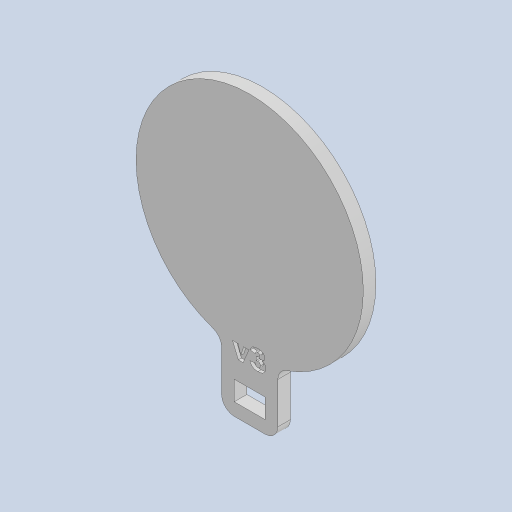
# Autodesk Inventor part: door_03
Saved by Autodesk Inventor 2024.4 (Build 284460030, 460C)
## iProperties
Created: 2026-07-13
Part Number: door_03
Material: Generic
Document SubType Name: Modeling
Designer: tooles01
Density: 1 g/cm^3
Appearance: Default
d0: 36.000 mm
d3: 4.900 mm
d4: 3.200 mm
d5: 10.000 mm
d6: 2.000 mm
d7: 2.000 mm
door_diameter: 36.000 mm
handle_height: 10.000 mm
spacing_height: 2.000 mm
spacing_width: 2.000 mm
axle_height: 3.100 mm
axle_width: 4.900 mm
x_e1: 0.00 deg
door_thickness: 2.000 mm
Author: tooles01
Autodesk Inventor part; units mm, degrees
ref_plane "YZ Plane" through (0, 0, 0) normal (1, 0, 0) x (0, 1, 0)
ref_plane "XZ Plane" through (0, 0, 0) normal (0, 1, 0) x (-1, 0, 0)
ref_plane "XY Plane" through (0, 0, 0) normal (0, 0, 1) x (1, 0, 0)
sketch "Sketch1: base" plane through (0, 0, 0) normal (0, 0, 1) x (1, 0, 0)
  circle A0 centre (0, 0) radius 18
  line L0 (4.45, -17.4413) -> (4.45, -27.4413)
  line L1 (4.45, -27.4413) -> (-4.45, -27.4413)
  line L2 (-4.45, -27.4413) -> (-4.45, -17.4413)
  line L3 (-2.45, -22.3413) -> (2.45, -22.3413)
  line L4 (2.45, -22.3413) -> (2.45, -25.4413)
  line L5 (2.45, -25.4413) -> (-2.45, -25.4413)
  line L6 (-2.45, -25.4413) -> (-2.45, -22.3413)
  line L7 (-2, -22.2913) -> (2, -22.2913) construction
  line L8 (2, -25.4913) -> (-2, -25.4913) construction
  arc A1 (-2, -22.2913) -> (-2, -25.4913) centre (-0.0791, -23.8913) ccw construction
  arc A2 (2, -25.4913) -> (2, -22.2913) centre (0.0791, -23.8913) ccw construction
  point P0 (0, -22.3413)
  point P1 (0, -27.4413)
  point P2 (0, -22.2913)
  point P3 (-2.45, -23.8913)
  dimension "door_diameter" = 36
  dimension "axle_width" = 4.9
  dimension "axle_height" = 3.1
  dimension "handle_height" = 10
  dimension "spacing_height" = 2
  dimension "spacing_width" = 2
  dimension "d14" = 4
  dimension "d16" = 3.2
  dimension "d17" = 2.5
  constraints: 18 end point, 6 point on circle, 5 perpendicular, 5 vertical alignment, 4 midpoint, 3 centre point, 3 horizontal, 1 coincident, 1 equal radius, 1 horizontal alignment
  measures "door_diameter" diameter of A0
  measures "axle_width" distance of L4.end L5.end
  measures "axle_height" distance of L5.end L3.start
  measures "handle_height" distance of L1.end L2.end
  measures "spacing_height" distance between parallel lines of L1 L5
  measures "spacing_width" distance between parallel lines of L2 L6
  measures "d14" distance of L7.start L7.end
  measures "d16" distance between parallel lines of L8 L7
  measures "d17" radius of A1
sketch "Sketch2: text" plane through (0, 0, 0) normal (0, 0, 1) x (1, 0, 0)
  line L0 (-1.5, -16.3413) -> (1.5, -16.3413) construction
  line L1 (1.5, -16.3413) -> (1.5, -19.3413) construction
  line L2 (1.5, -19.3413) -> (-1.5, -19.3413) construction
  line L3 (-1.5, -19.3413) -> (-1.5, -16.3413) construction
  line L4 (4.45, -27.4413) -> (-4.45, -27.4413) construction
  line L5 (-4.45, -27.4413) -> (-4.45, -17.4413) construction
  line L6 (4.45, -17.4413) -> (4.45, -27.4413) construction
  line L7 (-2.45, -22.3413) -> (2.45, -22.3413) construction
  line L8 (2.45, -22.3413) -> (2.45, -25.4413) construction
  line L9 (-2.45, -25.4413) -> (-2.45, -22.3413) construction
  line L10 (2.45, -25.4413) -> (-2.45, -25.4413) construction
  circle A0 centre (0, 0) radius 18 construction
  line L11 (-2.7183, -17.1558) -> (-1.8376, -17.1558)
  line L12 (-1.8376, -17.1558) -> (-1.4061, -18.5561)
  line L13 (-1.4061, -18.5561) -> (-0.9628, -17.1558)
  line L14 (-0.9628, -17.1558) -> (-0.1086, -17.1558)
  line L15 (-0.1086, -17.1558) -> (-1.048, -19.3663)
  line L16 (-1.048, -19.3663) -> (-1.7995, -19.3663)
  line L17 (-1.7995, -19.3663) -> (-2.7183, -17.1558)
  line L18 (0.8777, -17.1969) -> (0.0763, -17.0531)
  spline S0 degree 2 poles (0.0763, -17.0531) (0.1761, -16.6715) (0.7427, -16.2634) (1.2623, -16.2634) knots 0 0 0 1 2 2 2
  spline S1 degree 2 poles (1.2623, -16.2634) (1.8611, -16.2634) (2.3924, -16.7096) (2.3924, -17.0443) knots 0 0 0 1 2 2 2
  spline S2 degree 2 poles (2.3924, -17.0443) (2.3924, -17.2439) (2.1752, -17.5639) (1.9551, -17.6842) knots 0 0 0 1 2 2 2
  spline S3 degree 2 poles (1.9551, -17.6842) (2.1341, -17.7282) (2.2281, -17.787) knots 0 0 0 1 1 1
  spline S4 degree 2 poles (2.2281, -17.787) (2.3807, -17.8809) (2.548, -18.1862) (2.548, -18.3975) knots 0 0 0 1 2 2 2
  spline S5 degree 2 poles (2.548, -18.3975) (2.548, -18.6647) (2.2692, -19.1549) (1.7466, -19.4191) (1.318, -19.4191) knots 0 0 0 1 2 3 3 3
  spline S6 degree 2 poles (1.318, -19.4191) (0.9041, -19.4191) (0.4227, -19.2224) (0.1115, -18.8467) (0.0294, -18.5619) knots 0 0 0 1 2 3 3 3
  line L19 (0.0294, -18.5619) -> (0.8777, -18.4504)
  spline S7 degree 2 poles (0.8777, -18.4504) (0.9276, -18.7058) (1.136, -18.9024) (1.2975, -18.9024) knots 0 0 0 1 2 2 2
  spline S8 degree 2 poles (1.2975, -18.9024) (1.4678, -18.9024) (1.6938, -18.6529) (1.6938, -18.4445) knots 0 0 0 1 2 2 2
  spline S9 degree 2 poles (1.6938, -18.4445) (1.6938, -18.2302) (1.4766, -17.9983) (1.2887, -17.9983) knots 0 0 0 1 2 2 2
  spline S10 degree 2 poles (1.2887, -17.9983) (1.1889, -17.9983) (1.0157, -18.0482) knots 0 0 0 1 1 1
  line L20 (1.0157, -18.0482) -> (1.0597, -17.4406)
  spline S11 degree 2 poles (1.0597, -17.4406) (1.1302, -17.4523) (1.1683, -17.4523) knots 0 0 0 1 1 1
  spline S12 degree 2 poles (1.1683, -17.4523) (1.3357, -17.4523) (1.5588, -17.2409) (1.5588, -17.0942) knots 0 0 0 1 2 2 2
  spline S13 degree 2 poles (1.5588, -17.0942) (1.5588, -16.9562) (1.3914, -16.7889) (1.2476, -16.7889) knots 0 0 0 1 2 2 2
  spline S14 degree 2 poles (1.2476, -16.7889) (1.0979, -16.7889) (0.91, -16.9709) (0.8777, -17.1969) knots 0 0 0 1 2 2 2
  point P0 (0, -19.3413)
  point P1 (0, -22.3413)
  dimension "x_t2" = 3
  dimension "x_t3" = 3
  constraints: 2 midpoint, 1 horizontal, 1 perpendicular, 1 vertical alignment, 2 other
  measures "x_t2" distance of L0.start L0.end
  measures "x_t3" distance between parallel lines of L2 L7
extrude "Ex1: base" add sketch "Sketch1: base" against normal blind 2
extrude "Ex2: text" cut sketch "Sketch2: text" against normal blind 0.5
fillet "Fillet1" radius 2 4 edges at (4.45, -17.4413, -1) (-4.45, -17.4413, -1) (4.45, -27.4413, -1) (-4.45, -27.4413, -1)
fillet "Fillet2" [suppressed]
body "Solid1"
